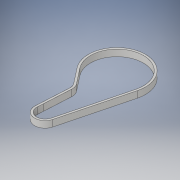
# Autodesk Inventor part: belt x
Saved by Autodesk Inventor 2019 (Build 230136000, 136)
## iProperties
Created: 2018-08-04
Part Number: belt x
Material: Generic
Document SubType Name: Modeling
Designer: torba
Density: 1 g/cm^3
Appearance: Default
Author: torba
Autodesk Inventor part; units mm, degrees
ref_plane "YZ Plane" through (0, 0, 0) normal (1, 0, 0) x (0, 1, 0)
ref_plane "XZ Plane" through (0, 0, 0) normal (0, 1, 0) x (-1, 0, 0)
ref_plane "XY Plane" through (0, 0, 0) normal (0, 0, 1) x (1, 0, 0)
sketch "Sketch1" plane through (0, 0, 0) normal (0, 1, 0) x (-1, 0, 0)
  arc A0 (68.1828, -106.1647) -> (70.806, -114.5442) centre (80.6635, -106.858) ccw
  arc A1 (15.8577, -154.8974) -> (86.8793, -140.1426) centre (55, -165) ccw
  line L0 (70.9754, -55.8873) -> (68.1828, -106.1647)
  line L1 (70.806, -114.5442) -> (89.2964, -138.2579)
  line L2 (67.3928, -65.1202) -> (65.1225, -105.9948)
  line L3 (68.3889, -116.4289) -> (86.8793, -140.1426)
  line L4 (39.5077, -51.0015) -> (12.89, -154.1315)
  line L5 (15.8577, -154.8974) -> (42.4754, -51.7674)
  arc A2 (70.9754, -55.8873) -> (39.5077, -51.0015) centre (55, -55) ccw
  arc A3 (70.9754, -55.8873) -> (39.5077, -51.0015) centre (55, -55) ccw construction
  arc A4 (12.89, -154.1315) -> (89.2964, -138.2579) centre (55, -165) ccw
  arc A5 (64.2134, -122.4869) -> (64.2065, -122.4854) centre (55, -165) ccw construction
  arc A6 (12.89, -154.1315) -> (89.2964, -138.2579) centre (55, -165) ccw
  arc A7 (65.1225, -105.9948) -> (68.3889, -116.4289) centre (80.6635, -106.858) ccw
  line L6 (67.3928, -65.1202) -> (67.9045, -55.8873)
  arc A8 (67.9045, -55.8873) -> (42.4754, -51.7674) centre (55, -55) ccw
  arc A9 (64.2134, -122.4869) -> (64.2065, -122.4854) centre (55, -165) ccw
  point P0 (0, 0)
  point P1 (68.1637, -106.913)
  point P2 (70.1289, -113.5865)
  constraints: 22 point on circle, 14 end point, 12 tangent, 10 centre point, 4 coincident, 2 parallel, 2 point on line, 1 concentric
extrude "Extrusion1" add sketch "Sketch1" along normal blind 10
equation "\"d12\" = -d2 + d1 + d0"
equation "\"d2\" = 25.87"
equation "\"d1\" = 32"
equation "\"d0\" = 25"
body "Solid1"
